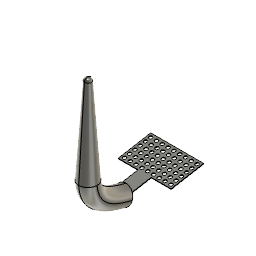
蒼角 _つの_mak1 v10 (Autodesk Fusion 360 design; units mm, degrees)
Autodesk Fusion 360 part; units mm, degrees
sketch "スケッチ1" plane through (0, 0, 0) normal (0, 0, 1) x (1, 0, 0)
  circle A0 centre (0, 0) radius 14
  dimension "d1" = 28
  constraint coincident A0.centre origin
  measures "d1" diameter of A0
ref_plane "作業平面2" through (0, 0, 135) normal (0, 0, 1) x (1, 0, 0)
sketch "スケッチ4" plane through (0, 0, 135) normal (0, 0, 1) x (1, 0, 0)
  circle A0 centre (0, 0) radius 5
  dimension "d15" = 10
  constraint coincident A0.centre origin
  measures "d15" diameter of A0
loft "ロフト1" add profiles "スケッチ1", "スケッチ4" section 1 section 2 makes body 1
sketch "スケッチ7" plane through (0, 0, 0) normal (1, 0, 0) x (0, 1, 0)
  spline S0 degree 5 poles (0, 0) (0.1251, -1.4441) (0.4611, -4.2841) (1.2223, -8.3999) (2.7601, -13.5946) (5.6092, -19.5683) (9.454, -24.9838) (14.3525, -29.8086) (20.2964, -34.0473) (27.2092, -37.7428) (35.0009, -40.9456) (41.872, -43.1503) (47.36, -44.6162) (51.165, -45.5114) (53.1041, -45.9385) knots 0 0 0 0 0 0 0.1 0.2 0.3 0.4 0.5 0.6 0.7 0.8 0.9 1 1 1 1 1 1
  point P0 (12.046, -27.3341)
  constraint coincident S0.start origin
sweep "スイープ1" add 1 faces at (4.6394, 2.5701, 0) path "スケッチ7" along S0 on bodies 1 bodies 1
fillet "フィレット1" radius 5 1 edges at (-4.6616, 1.8081, 135) on bodies 1
sketch "スケッチ8" plane through (0, 61.4607, -19.2292) normal (0, 0.954379, -0.298597) x (-1, 0, 0)
  circle A0 centre (0, -27.986) radius 14
  line L0 (-10, -19.486) -> (10, -19.486)
  line L1 (10, -19.486) -> (10, -20.986)
  line L2 (10, -20.986) -> (-10, -20.986)
  line L3 (-10, -20.986) -> (-10, -19.486)
  line L4 (0, -27.986) -> (0, -20.986)
  dimension "d18" = 20
  dimension "d20" = 1.5
  dimension "d21" = 7
  constraint horizontal L0
  constraint vertical L1
  constraint horizontal L2
  constraint vertical L3
  constraint coincident A0.centre L4.start
  constraint coincident L2 L4.end
  constraint perpendicular L2 L4
  constraint midpoint L2 L4.end
  measures "d18" distance of L0.start L0.end
  measures "d20" distance of L0.end L1.end
  measures "d21" distance of A0.centre L4.end
ref_plane "作業平面3" through (0, 55.6422, -37.8263) normal (0, 0.984808, 0.173648) x (-1, 0, 0)
sketch "スケッチ15" plane through (0, 47.4957, 8.3748) normal (0, 0.984808, 0.173648) x (-1, 0, 0)
  line L0 (-10, -47) -> (10, -47)
  line L1 (10, -47) -> (10, -50)
  line L2 (10, -50) -> (-10, -50)
  line L3 (-10, -50) -> (-10, -47)
  constraint horizontal L0
  constraint vertical L1
  constraint horizontal L2
  constraint vertical L3
extrude "押し出し8" cut sketch "スケッチ15" against normal blind 30 bodies 1
sketch "スケッチ16" plane through (0, 8.1615, -46.286) normal (0, 0.173648, -0.984808) x (-1, 0, 0)
  line L0 (10, 48.1838) -> (-10, 48.1838)
  line L1 (-10, 48.1838) -> (-10, 18.2284)
  line L2 (-10, 18.2284) -> (10, 18.2284)
  line L3 (10, 18.2284) -> (10, 48.1838)
  line L4 (0, 48.1838) -> (0, 38.1838)
  circle A0 centre (0, 38.1838) radius 4
  circle A1 centre (0, 38.1838) radius 2.75
  dimension "d64" = 10
  dimension "d65" = 8
  dimension "d66" = 5.5
  constraint midpoint L0 L4.start
  constraint perpendicular L0 L4
  constraint coincident L4.end A0.centre
  constraint concentric A0 A1
  measures "d64" distance of L4.start L4.end
  measures "d65" diameter of A0
  measures "d66" diameter of A1
sketch "スケッチ17" plane through (0, 17.9514, 3.1653) normal (0, 0.984808, 0.173648) x (-1, 0, 0)
  line L0 (-10, -50) -> (10, -50)
  line L1 (10, -50) -> (10, -47)
  line L2 (10, -47) -> (-10, -47)
  line L3 (-10, -47) -> (-10, -50)
  line L4 (-10, -47) -> (10, -47)
  line L5 (10, -47) -> (10, -49.5)
  line L6 (10, -49.5) -> (-10, -49.5)
  line L7 (-10, -49.5) -> (-10, -47)
  dimension "d71" = 2.5
  constraint horizontal L4
  constraint vertical L5
  constraint horizontal L6
  constraint vertical L7
  constraint coincident L2.end L3.start
  measures "d71" distance of L2.end L6.end
extrude "押し出し12" add sketch "スケッチ17" along normal blind 30 separate body contours L1 L2 L3 L4 L5 L6 L7 makes body 2
split "分割2" by plane through (0, 0, 0) normal (1, 0, 0) bodies 1 makes body 3 at (12.4259, 5.3211, 7.2407)
sketch "スケッチ20" plane through (0, 47.4957, 8.3748) normal (0, 0.984808, 0.173648) x (-1, 0, 0)
  line L0 (-10, -49.5) -> (10, -49.5)
  line L1 (10, -49.5) -> (10, -47)
  line L2 (10, -47) -> (-10, -47)
  line L3 (-10, -47) -> (-10, -49.5)
  line L4 (-10, -49.5) -> (10, -49.5)
  line L5 (10, -49.5) -> (10, -48.5)
  line L6 (10, -48.5) -> (-10, -48.5)
  line L7 (-10, -48.5) -> (-10, -49.5)
  dimension "d78" = 1
  constraint horizontal L4
  constraint vertical L5
  constraint horizontal L6
  constraint vertical L7
  constraint coincident L0.start L3.end
  measures "d78" distance of L0.start L6.end
extrude "押し出し14" add sketch "スケッチ20" along normal blind 80 contours L0 L1 L3 L4 L5 L6 L7 bodies 2
sketch "スケッチ21" plane through (10, 0, 0) normal (1, 0, 0) x (0, 1, 0)
  line L0 (26.1129, -43.1206) -> (26.547, -45.5827)
  line L1 (26.547, -45.5827) -> (134.8759, -26.4814)
  line L2 (134.8759, -26.4814) -> (134.7022, -25.4966)
  line L3 (134.7022, -25.4966) -> (55.9176, -39.3884)
  line L4 (55.9176, -39.3884) -> (55.6571, -37.9112)
  line L5 (55.6571, -37.9112) -> (26.1129, -43.1206)
  line L6 (134.8759, -26.4814) -> (85.6355, -35.1638)
  line L7 (85.6355, -35.1638) -> (85.4619, -34.179)
  line L8 (85.4619, -34.179) -> (134.7022, -25.4966)
  line L9 (134.7022, -25.4966) -> (134.8759, -26.4814)
  dimension "d81" = 50
  constraint coincident L1.end L2.start
  constraint perpendicular L2 L6
  constraint coincident L3 L7.end
  constraint perpendicular L3 L7
  constraint coincident L2.end L3.start
  measures "d81" distance of L1.end L6.end
extrude "押し出し15" add sketch "スケッチ21" along normal blind 30 separate body contours L1 L2 L3 L6 L7 L8 L9 makes body 4
mirror "ミラー1" about plane through (0, 0, 0) normal (1, 0, 0) of bodies 4 makes body 5
combine "結合1" operation add target body 4 tool bodies 2 5
sketch "スケッチ22" plane through (0, 8.4219, -47.7632) normal (0, -0.173648, 0.984808) x (1, 0, 0)
  line L0 (10, 78.2284) -> (40, 78.2284)
  line L1 (40, 78.2284) -> (40, 128.2284)
  line L2 (40, 128.2284) -> (-40, 128.2284)
  line L3 (-40, 128.2284) -> (-40, 78.2284)
  line L4 (-40, 78.2284) -> (-10, 78.2284)
  line L5 (-10, 78.2284) -> (-10, 48.2284)
  line L6 (-10, 48.2284) -> (10, 48.2284)
  line L7 (10, 48.2284) -> (10, 78.2284)
  circle A0 centre (0, 83) radius 2.5
  circle A1 centre (0, 91) radius 2.5
  circle A2 centre (0, 99) radius 2.5
  circle A3 centre (0, 107) radius 2.5
  circle A4 centre (0, 115) radius 2.5
  circle A5 centre (0, 123) radius 2.5
  circle A6 centre (-35, 83) radius 2.5
  circle A7 centre (-35, 115) radius 2.5
  circle A8 centre (-35, 123) radius 2.5
  circle A9 centre (-35, 107) radius 2.5
  circle A10 centre (-35, 99) radius 2.5
  circle A11 centre (-35, 91) radius 2.5
  circle A12 centre (-26.25, 83) radius 2.5
  circle A13 centre (-26.25, 115) radius 2.5
  circle A14 centre (-26.25, 123) radius 2.5
  circle A15 centre (-26.25, 107) radius 2.5
  circle A16 centre (-26.25, 99) radius 2.5
  circle A17 centre (-26.25, 91) radius 2.5
  circle A18 centre (-17.5, 83) radius 2.5
  circle A19 centre (-17.5, 115) radius 2.5
  circle A20 centre (-17.5, 123) radius 2.5
  circle A21 centre (-17.5, 107) radius 2.5
  circle A22 centre (-17.5, 99) radius 2.5
  circle A23 centre (-17.5, 91) radius 2.5
  circle A24 centre (-8.75, 83) radius 2.5
  circle A25 centre (-8.75, 115) radius 2.5
  circle A26 centre (-8.75, 123) radius 2.5
  circle A27 centre (-8.75, 107) radius 2.5
  circle A28 centre (-8.75, 99) radius 2.5
  circle A29 centre (-8.75, 91) radius 2.5
  circle A30 centre (8.75, 83) radius 2.5
  circle A31 centre (8.75, 115) radius 2.5
  circle A32 centre (8.75, 123) radius 2.5
  circle A33 centre (8.75, 107) radius 2.5
  circle A34 centre (8.75, 99) radius 2.5
  circle A35 centre (8.75, 91) radius 2.5
  circle A36 centre (17.5, 83) radius 2.5
  circle A37 centre (17.5, 115) radius 2.5
  circle A38 centre (17.5, 123) radius 2.5
  circle A39 centre (17.5, 107) radius 2.5
  circle A40 centre (17.5, 99) radius 2.5
  circle A41 centre (17.5, 91) radius 2.5
  circle A42 centre (26.25, 83) radius 2.5
  circle A43 centre (26.25, 115) radius 2.5
  circle A44 centre (26.25, 123) radius 2.5
  circle A45 centre (26.25, 107) radius 2.5
  circle A46 centre (26.25, 99) radius 2.5
  circle A47 centre (26.25, 91) radius 2.5
  circle A48 centre (35, 83) radius 2.5
  circle A49 centre (35, 115) radius 2.5
  circle A50 centre (35, 123) radius 2.5
  circle A51 centre (35, 107) radius 2.5
  circle A52 centre (35, 99) radius 2.5
  circle A53 centre (35, 91) radius 2.5
  dimension "d86" = 5
  dimension "d89" = 0
  dimension "d90" = 40
  dimension "d93" = 35
  dimension "d94" = 0
  measures "d86" diameter of A0
extrude "押し出し16" cut sketch "スケッチ22" against normal blind 7 contours A0 | A1 | A2 | A3 | A4 | A5 | A6 | A7 | A8 | A9 | A10 | A11 | A12 | A13 | A14 | A15 | A16 | A17 | A18 | A19 | A20 | A21 | A22 | A23 | A24 | A25 | A26 | A27 | A28 | A29 | A30 | A31 | A32 | A33 | A34 | A35 | A36 | A37 | A38 | A39 | A40 | A41 | A42 | A43 | A44 | A45 | A46 | A47 | A48 | A49 | A50 | A51 | A52 | A53 bodies 4
fillet "フィレット2" radius 1 1 edges at (0, 55.9176, -39.3884) on bodies 4
